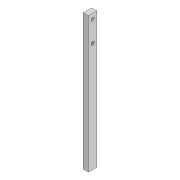
# Autodesk Inventor part: Vertical_bar
Saved by Autodesk Inventor 2022 (Build 260153000, 153)
## iProperties
Created: 2022-08-23
Part Number: Vertical_bar
Material: Generic
Document SubType Name: Modeling
Designer: dell
Density: 1 g/cm^3
Appearance: Default
Mass: 6.42931 g
Surface Area: 40.6597 cm^2
Volume: 6.42931 cm^3
Author: dell
Autodesk Inventor part; units mm, degrees
ref_plane "YZ Plane" through (0, 0, 0) normal (1, 0, 0) x (0, 1, 0)
ref_plane "XZ Plane" through (0, 0, 0) normal (0, 1, 0) x (-1, 0, 0)
ref_plane "XY Plane" through (0, 0, 0) normal (0, 0, 1) x (1, 0, 0)
sketch "Sketch1" plane through (0, 0, 0) normal (1, 0, 0) x (0, 1, 0)
  line L0 (0, 0) -> (130, 0)
  line L1 (130, 0) -> (130, -8)
  line L2 (130, -8) -> (0, -8)
  line L3 (0, -8) -> (0, 0)
  circle A0 centre (125, -4) radius 1.5
  circle A1 centre (105, -4) radius 1.5
  dimension "d0" = 130
  dimension "d1" = 8
  dimension "d4" = 3
  dimension "d5" = 5
  dimension "d6" = 3
  dimension "d8" = 20
  dimension "d9" = 4
  dimension "d10" = 4
  constraints: 8 end point, 2 centre point, 2 parallel, 1 horizontal, 1 perpendicular
  measures "d0" distance of L1.end L2.end
  measures "d1" distance between parallel lines of L0 L2
  measures "d4" diameter of A0
  measures "d5" distance from line of L1 A0.centre
  measures "d6" diameter of A1
  measures "d8" distance of A1.centre A0.centre
  measures "d9" vertical distance of L0.end A0.centre
  measures "d10" distance from line of L0 A1.centre
extrude "Extrusion1" add sketch "Sketch1" along normal blind 5
equation "\"d9\" = 0.5 * d1"
equation "\"d10\" = 0.5 * d1"
body "Solid1"
